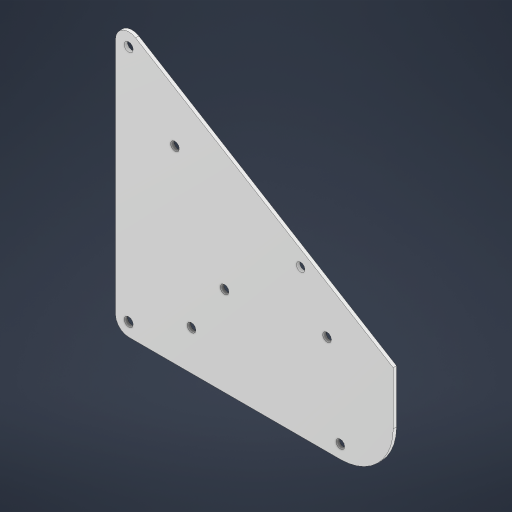
# Autodesk Inventor part: blocker
Saved by Autodesk Inventor 2024 (Build 280153000, 153)
## iProperties
Created: 2023-11-29
Part Number: blocker
Material: Acetal Resin, White
Document SubType Name: Modeling
Designer: avere
Density: 1.425 g/cm^3
Appearance: Smooth - White
Author: avere
Autodesk Inventor part; units mm, degrees
ref_plane "YZ Plane" through (0, 0, 0) normal (1, 0, 0) x (0, 1, 0)
ref_plane "XZ Plane" through (0, 0, 0) normal (0, 1, 0) x (-1, 0, 0)
ref_plane "XY Plane" through (0, 0, 0) normal (0, 0, 1) x (1, 0, 0)
sketch "Sketch1" plane through (0, 0, 0) normal (0, 0, 1) x (1, 0, 0)
  circle A0 centre (-64.8392, -51.6694) radius 2.1844
  circle A1 centre (-64.8392, 62.6306) radius 2.1844
  arc A2 (-71.1892, -51.6694) -> (-64.8392, -58.0194) centre (-64.8392, -51.6694) ccw
  arc A3 (-61.5382, 68.0552) -> (-71.1892, 62.6306) centre (-64.8392, 62.6306) ccw
  line L0 (-64.8392, -58.0194) -> (36.7608, -58.0194)
  line L1 (62.1608, -32.6194) -> (62.1608, -7.2194)
  line L2 (62.1608, -7.2194) -> (-61.5382, 68.0552)
  arc A4 (36.7608, -58.0194) -> (62.1608, -32.6194) centre (36.7608, -32.6194) ccw
  line L3 (-71.1892, -51.6694) -> (-71.1892, 62.6306)
  circle A5 centre (36.7608, -51.6694) radius 2.0955
  circle A6 centre (30.4108, -10.3944) radius 2.0955
  circle A7 centre (-34.6767, -38.9694) radius 2.0955
  circle A8 centre (17.7108, 12.3965) radius 2.0955
  circle A9 centre (-18.8017, -15.1569) radius 2.0955
  circle A10 centre (-42.6142, 32.4681) radius 2.0955
  point P0 (0, 0)
  point P1 (62.1608, -58.0194)
  dimension "d0" = 12.7
  dimension "d1" = 12.7
  dimension "d2" = 50.8
  dimension "d3" = 25.4
  dimension "d4" = 4.191
  dimension "d5" = 4.191
  dimension "d6" = 4.191
  dimension "d7" = 4.191
  dimension "d8" = 4.191
  dimension "d9" = 4.191
  constraints: 11 centre point, 8 end point, 6 point on circle, 4 tangent, 2 coincident, 2 point on line, 1 horizontal, 1 perpendicular
  measures "d0" diameter of A2
  measures "d1" diameter of A3
  measures "d2" distance of point (62.161, -58.019) L2.start
  measures "d3" radius of A4
  measures "d4" diameter of A5
  measures "d5" diameter of A6
  measures "d6" diameter of A7
  measures "d7" diameter of A8
  measures "d8" diameter of A9
  measures "d9" diameter of A10
extrude "Extrusion1" add sketch "Sketch1" along normal blind 1.5875
body "Solid1"
